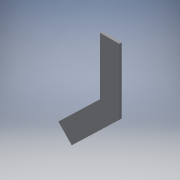
# Autodesk Inventor part: bottom gusset
Saved by Autodesk Inventor 2016 (Build 200138000, 138)
## iProperties
Created: 2016-02-23
Part Number: bottom gusset
Material: Aluminum 6061
Document SubType Name: Modeling
Designer: gus
Density: 2.7 g/cm^3
Appearance: Aluminum - Flat
Author: gus
Autodesk Inventor part; units mm, degrees
ref_plane "YZ Plane" through (0, 0, 0) normal (1, 0, 0) x (0, 1, 0)
ref_plane "XZ Plane" through (0, 0, 0) normal (0, 1, 0) x (-1, 0, 0)
ref_plane "XY Plane" through (0, 0, 0) normal (0, 0, 1) x (1, 0, 0)
sketch "Sketch1" plane through (0, 0, 0) normal (0, 0, 1) x (1, 0, 0)
  line L0 (0, 0) -> (-62.6699, -60.3488)
  line L1 (0, 0) -> (0, 87.0028)
  line L2 (0, 87.0028) -> (-25.4, 87.0028)
  line L3 (-25.4, 87.0028) -> (-25.4, 10.8028)
  line L4 (-25.4, 10.8028) -> (-80.2884, -42.0527)
  line L5 (-80.2884, -42.0527) -> (-62.6699, -60.3488)
  dimension "d0" = 25.4
  dimension "d1" = 76.2
  dimension "d2" = 133.919
  constraints: 12 end point, 3 perpendicular, 2 equal length, 1 horizontal, 1 vertical
  measures "d0" distance of L1.end L2.end
  measures "d1" distance of L2.end L3.end
  measures "d2" angle of L4 L3
extrude "Extrusion1" add sketch "Sketch1" along normal blind 3.175
body "Solid1"
